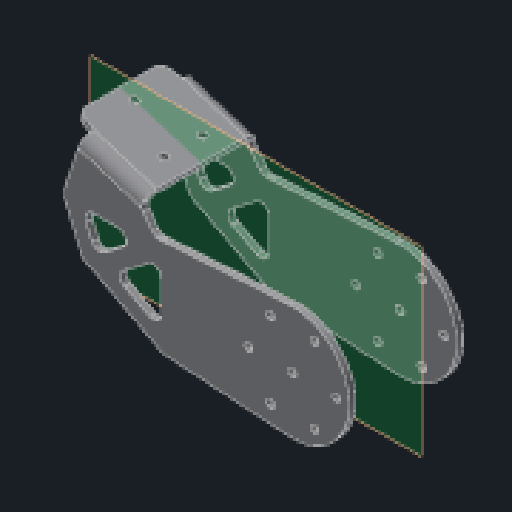
# Autodesk Inventor part: Hip
Saved by Autodesk Inventor 2025.2 (Build 292293000, 293)
## iProperties
Created: 2020-05-23
Part Number: Hip
Material: Generic
Document SubType Name: Sheet Metal
Designer: valer
Density: 1 g/cm^3
Sheet Metal Rule: Default
Appearance: Default
Author: valer
Autodesk Inventor part; units mm, degrees
ref_plane "YZ Plane" through (0, 0, 0) normal (1, 0, 0) x (0, 1, 0)
ref_plane "XZ Plane" through (0, 0, 0) normal (0, 1, 0) x (-1, 0, 0)
ref_plane "XY Plane" through (0, 0, 0) normal (0, 0, 1) x (1, 0, 0)
sketch "Base" plane through (0, 0, 0) normal (0, 0, 1) x (1, 0, 0)
  circle A0 centre (0, 0) radius 44.7044
  circle A1 centre (0, 0) radius 3.175
  circle A2 centre (-17.2777, 29.9259) radius 3.175
  circle A3 centre (-34.5555, 0) radius 3.175
  circle A4 centre (-17.2777, -29.9259) radius 3.175
  circle A5 centre (17.2777, -29.9259) radius 3.175
  circle A6 centre (34.5555, 0) radius 3.175
  circle A7 centre (17.2777, 29.9259) radius 3.175
  line L0 (0, 0) -> (-101.6, 0) construction
  circle A8 centre (0, 0) radius 34.5555 construction
  line L1 (0, 0) -> (17.2777, 29.9259) construction
  line L2 (0, 0) -> (-17.2777, 29.9259) construction
  line L3 (0, 0) -> (-34.5555, 0) construction
  line L4 (0, 0) -> (34.5555, 0) construction
  line L5 (0, 0) -> (17.2777, -29.9259) construction
  line L6 (0, 0) -> (-17.2777, -29.9259) construction
  line L7 (-2.9423, 44.6075) -> (-101.6, 38.1)
  line L8 (-2.9423, -44.6075) -> (-101.6, -38.1)
  line L9 (-101.6, 38.1) -> (-101.6, -38.1) construction
  line L10 (-101.6, -38.1) -> (-187.4356, 7.5396)
  line L11 (-187.4356, 7.5396) -> (-177.8, 38.1)
  line L12 (-177.8, 38.1) -> (-101.6, 38.1)
  line L13 (-177.8, 38.1) -> (-168.2526, 68.3805)
  line L14 (-168.2526, 68.3805) -> (-119.0864, 52.8785)
  line L15 (-119.0864, 52.8785) -> (-107.95, 38.1)
  dimension "d0" = 89.4088
  dimension "d2" = 6.35
  dimension "d4" = 101.6
  dimension "d5" = 69.111
  dimension "d6" = 60
  dimension "d7" = 60
  dimension "d8" = 60
  dimension "d9" = 60
  dimension "d10" = 60
  dimension "d11" = 60
  dimension "d15" = 62
  dimension "d16" = 100.5
  dimension "d18" = 76.2
  dimension "d26" = 76.2
  dimension "d27" = 53
  dimension "d28" = 6.35
  dimension "d29" = 31.75
  dimension "d85" = 176.226
  measures "d0" diameter of A0
  measures "d2" diameter of A2
  measures "d4" distance of L0.end L0.start
  measures "d5" diameter of A8
  measures "d6" angle of L1 L2
  measures "d7" angle of L4 L1
  measures "d8" angle of L5 L4
  measures "d9" angle of L5 L6
  measures "d10" angle of L3 L6
  measures "d11" angle of L2 L3
  measures "d15" angle of L9 L10
  measures "d16" angle of L10 L11
  measures "d18" distance of L11.end L7.end
  measures "d26" distance of L7.end L8.end
  measures "d27" angle of L12 L15
  measures "d28" distance of L7.end L15.end
  measures "d29" distance of L11.end L13.end
  measures "d85" angle of L7 L12
extrude "Plate1" add sketch "Base" along normal blind 5
sketch "Sketch4" plane through (-117.5828, 57.647, -5) normal (0.3007058, 0.953717, 0) x (-0.953717, 0.3007058, 0)
  line L0 (51.5522, 0) -> (0, 0)
  line L1 (0, 0) -> (0, -34.58)
  line L2 (0, -34.58) -> (51.5522, -34.58)
  line L3 (51.5522, -34.58) -> (51.5522, 0)
  constraints: 6 end point, 1 horizontal, 1 perpendicular, 1 vertical
edge flange "MountFlangeFeature" height 44.58 angle 90 thickness 5 bend radius 5 thickness toward (0.3007058, 0.953717, 0) relief straight relief width 5 relief depth 2.5 edges at (-143.6695, 60.6295, 0) wall of the first edge with corners at (-166.7491, 73.1491, -5) (-117.5828, 57.647, -5) (-117.5828, 57.647, -39.58) (-166.7491, 73.1491, -39.58)
bend "Bend1"
corner "Corner1"
chamfer "CornerChamferFeature" distance 25.4 angle 45 1 edges at (-187.4356, 7.5396, 2.5)
fillet "OutsideFilletsFeature" radius 6.35 5 edges at (-179.7977, 31.764, 2.5) (-165.0088, -4.385, 2.5) (-101.6, -38.1, 2.5) (-107.95, 38.1, 2.5) (-119.0864, 52.8785, 2.5)
sketch "GenerativeHoles" plane through (0, 0, 5) normal (0, 0, 1) x (1, 0, 0)
  line L0 (-102.8033, 25.293) -> (-102.8033, -23.0765)
  line L1 (-102.8033, -23.0765) -> (-140.4373, -3.0662)
  line L2 (-140.4373, -3.0662) -> (-102.8033, 25.293)
  line L3 (-154.1155, 2.5287) -> (-117.7163, 29.9574)
  line L4 (-117.7163, 29.9574) -> (-165.3369, 29.9574)
  line L5 (-165.3369, 29.9574) -> (-154.1155, 2.5287)
  line L6 (-117.1182, 50.2666) -> (-109.8553, 40.6285) projected
  line L7 (-102.8033, -37.4602) -> (-162.9819, -5.4626) projected
  line L8 (-165.878, -2.2603) -> (-178.9285, 29.6394) projected
  line L9 (-101.6, 38.1) -> (-2.9423, 44.6075) projected
  point P0 (0, 0)
  dimension "d75" = 12.7
  dimension "d76" = 12.7
  dimension "d77" = 12.7
  dimension "d78" = 12.7
  dimension "d79" = 12.7
  dimension "d80" = 0
  constraints: 12 end point, 3 parallel, 2 perpendicular, 1 vertical
  measures "d75" distance between parallel lines of L7 L1
  measures "d76" distance between parallel lines of L8 L5
  measures "d77" distance from line of L9 L0.start
  measures "d78" distance from line of L6 L3.end
  measures "d79" distance between parallel lines of L2 L3
  measures "d80" horizontal distance of L7.start L0.end
extrude "GenerativeHolesFeature" cut sketch "GenerativeHoles" against normal blind 25.4
fillet "GenerativeFilletsFeature" radius 6.35 6 edges at (-154.1155, 2.5287, 2.5) (-165.3369, 29.9574, 2.5) (-117.7163, 29.9574, 2.5) (-102.8033, 25.293, 2.5) (-140.4373, -3.0662, 2.5) (-102.8033, -23.0765, 2.5)
mirror "MirrorFeature" about plane through (-166.7491, 73.1491, -39.58) normal (0, 0, -1)
sketch "Mount" plane through (-165.2455, 77.9177, -5) normal (0.3007058, 0.953717, 0) x (0.953717, -0.3007058, 0)
  line L0 (0, 74.16) -> (0, 69.16)
  line L1 (0, 0) -> (0, 69.16)
  line L2 (0, 69.16) -> (0, 0)
  line L3 (0, 0) -> (-15, 3.075)
  line L4 (-15, 3.075) -> (-15, 66.085)
  line L5 (-15, 66.085) -> (0, 69.16)
  point P0 (181.0278, -5)
  dimension "d54" = 78.415
  dimension "d55" = 78.415
  dimension "d63" = 15
  measures "d54" angle of L1 L5
  measures "d55" angle of L1 L3
  measures "d63" distance between parallel lines of L4 L1
sheet face with bend "MountFeature" sketch "Mount" thickness 5 toward (-0.3007058, -0.953717, 0) bend radius 5 relief straight relief width 5 relief depth 2.5
bend "Bend2"
fillet "MountFilletsFeature" radius 6.35 2 edges at (-180.3031, 80.044, -8.075) (-180.3031, 80.044, -71.085)
sketch "MountHoles" plane through (-116.0793, 62.4156, -5) normal (0.3007058, 0.953717, 0) x (0.953717, -0.3007058, 0)
  line L0 (-66.5522, 60.9047) -> (-66.5522, 8.2553) construction
  line L1 (0, 69.16) -> (0, 0) construction
  line L2 (-66.5522, 60.9047) -> (-66.5522, 8.2553) construction
  line L3 (-66.5522, 34.58) -> (0, 34.58) construction
  line L4 (0, 69.16) -> (0, 0) construction
  line L5 (-14.5522, 19.58) -> (-14.5522, 49.58) construction
  circle A0 centre (-14.5522, 19.58) radius 3
  circle A1 centre (-14.5522, 49.58) radius 3
  circle A2 centre (-54.5522, 34.58) radius 3
  point P0 (129.4756, -5)
  point P1 (-14.5522, 34.58)
  dimension "d64" = 6
  dimension "d65" = 30
  dimension "d84" = 40
  dimension "d86" = 12
  constraints: 4 end point, 3 centre point, 3 midpoint, 2 coincident, 2 equal radius, 2 point on line, 1 vertical
  measures "d64" diameter of A0
  measures "d65" distance of L5.start L5.end
  measures "d84" distance from line of L5 A2.centre
  measures "d86" distance from line of L0 A2.centre
hole "MountHolesFeature" at (-129.958, 66.7916, -24.58) at (-168.1067, 78.8198, -39.58) at (-129.958, 66.7916, -54.58) direction (-0.3007058, -0.953717, 0) diameter 6.35 end through all
ref_plane "MidPlane" through (0, 0, -39.58) normal (0, 0, -1) x (-1, 0, 0)
equation "\"d55\" = d54"
equation "\"d73\" = Thickness"
equation "\"d14\" = Thickness"
equation "\"d30\" = BendReliefWidth"
equation "\"d31\" = BendReliefDepth"
equation "\"d32\" = MinimumRemnant"
equation "\"d33\" = TransitionRadius"
equation "\"d36\" = BendRadius"
equation "\"d37\" = CornerReliefSize"
equation "\"d38\" = GapSize"
equation "\"d39\" = JacobiRadiusSize"
equation "\"d57\" = BendRadius"
equation "\"d58\" = BendReliefWidth"
equation "\"d60\" = MinimumRemnant"
equation "\"d59\" = BendReliefDepth"
equation "\"d61\" = TransitionRadius"
equation "\"BendRadius\" = Thickness"
equation "\"BendReliefWidth\" = Thickness"
equation "\"BendReliefDepth\" = 0.5 * Thickness"
equation "\"TransitionRadius\" = BendRadius"
equation "\"JacobiRadiusSize\" = BendRadius"
equation "\"GapSize\" = Thickness"
equation "\"Thickness\" = 5"
equation "\"MinimumRemnant\" = 10"
equation "\"CornerReliefSize\" = 20"
body "Solid1"
